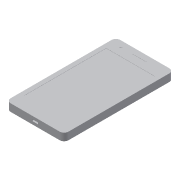
# Autodesk Inventor part: Galaxy S2
Saved by Autodesk Inventor 2013 (Build 170138000, 138)
## iProperties
Created: 2013-06-30
Part Number: Galaxy S2
Material: Allgemein
Document SubType Name: Modeling
Designer: Harald
Density: 1 g/cm^3
Author: Harald
Autodesk Inventor part; units mm, degrees
ref_plane "YZ Plane" through (0, 0, 0) normal (1, 0, 0) x (0, 1, 0)
ref_plane "XZ Plane" through (0, 0, 0) normal (0, 1, 0) x (-1, 0, 0)
ref_plane "XY Plane" through (0, 0, 0) normal (0, 0, 1) x (1, 0, 0)
sketch "Skizze1" plane through (0, 0, 0) normal (0, 0, 1) x (1, 0, 0)
  line L0 (0, 0) -> (66.1, 0)
  line L1 (66.1, 0) -> (66.1, 125.3)
  line L2 (66.1, 125.3) -> (0, 125.3)
  line L3 (0, 125.3) -> (0, 0)
  dimension "d0" = 66.1
  dimension "d1" = 125.3
  constraints: 8 end point, 2 parallel, 1 horizontal, 1 perpendicular
  measures "d0" distance of L2.end L1.end
  measures "d1" distance of L0.end L1.end
extrude "Extrusion1" add sketch "Skizze1" along normal blind 8.5
fillet "Rundung1" radius 5 1 edges at (66.1, 125.3, 4.25)
fillet "Rundung2" radius 5 1 edges at (0, 125.3, 4.25)
fillet "Rundung3" radius 5 1 edges at (0, 0, 4.25)
fillet "Rundung4" radius 5 1 edges at (66.1, 0, 4.25)
sketch "Skizze2" plane through (0, 0, 8.5) normal (0, 0, 1) x (1, 0, 0)
  line L0 (66.1, 5) -> (66.1, 120.3) projected
  line L1 (61.1, 125.3) -> (5, 125.3) projected
  line L2 (0, 120.3) -> (0, 5) projected
  line L3 (5.05, 109.15) -> (61.05, 109.15)
  line L4 (61.05, 109.15) -> (61.05, 16.15)
  line L5 (61.05, 16.15) -> (5.05, 16.15)
  line L6 (5.05, 16.15) -> (5.05, 109.15)
  point P0 (0, 0)
  dimension "d8" = 56
  dimension "d9" = 93
  dimension "d10" = 5.05
  dimension "d11" = 16.15
  constraints: 8 end point, 2 parallel, 1 horizontal, 1 perpendicular
  measures "d8" distance of L4.end L5.end
  measures "d9" distance of L3.end L4.end
  measures "d10" distance between parallel lines of L6 L2
  measures "d11" distance between parallel lines of L3 L1
sketch "Skizze3" plane through (0, 0, 8.5) normal (0, 0, 1) x (1, 0, 0)
  line L0 (66.1, 5) -> (66.1, 120.3) projected
  line L1 (61.1, 125.3) -> (5, 125.3) projected
  line L2 (0, 120.3) -> (0, 5) projected
  line L3 (5, 0) -> (61.1, 0) projected
  circle A0 centre (12, 118.6) radius 1.5
  line L4 (25.9, 119.7) -> (40.2, 119.7)
  arc A1 (40.2, 118.3) -> (40.2, 119.7) centre (40.2, 119) ccw
  line L5 (40.2, 118.3) -> (25.9, 118.3)
  arc A2 (25.9, 119.7) -> (25.9, 118.3) centre (25.9, 119) ccw
  point P0 (0, 0)
  dimension "d0" = 66.1
  dimension "d12" = 6.7
  dimension "d13" = 12
  dimension "d14" = 3
  dimension "d19" = 1.4
  dimension "d22" = 5.6
  dimension "d23" = 15.7
  dimension "d27" = 14.3
  dimension "d28" = 25.9
  constraints: 4 end point, 4 point on circle, 3 centre point, 2 parallel, 1 equal radius, 1 tangent, 1 vertical alignment
  measures "d12" distance from line of A0.centre L1
  measures "d13" distance from line of L2 A0.centre
  measures "d14" diameter of A0
  measures "d19" distance between parallel lines of L5 L4
  measures "d22" distance between parallel lines of L4 L1
  measures "d27" distance of A2.centre A1.centre
  measures "d28" distance from line of L0 A1.centre
extrude "Extrusion2" add sketch "Skizze3" along normal blind 0.2
extrude "Extrusion3" cut sketch "Skizze2" against normal blind 0.2
sketch "Skizze5" plane through (5, 0, 0) normal (0, -1, 0) x (1, 0, 0)
  line L0 (0, 8.5) -> (56.1, 8.5) projected
  line L1 (0, 0) -> (0, 8.5) projected
  line L2 (0, 0) -> (56.1, 0) projected
  line L3 (24.575, 5.15) -> (31.425, 5.15)
  line L4 (31.425, 5.15) -> (31.425, 3.35)
  line L5 (31.425, 3.35) -> (24.575, 3.35)
  line L6 (24.575, 3.35) -> (24.575, 5.15)
  line L7 (56.1, 8.5) -> (56.1, 0) projected
  line L8 (0, 8.5) -> (56.1, 8.5) projected
  line L9 (0, 0) -> (0, 8.5) projected
  line L10 (0, 0) -> (56.1, 0) projected
  point P0 (-5, 0)
  dimension "d33" = 6.85
  dimension "d34" = 1.8
  dimension "d35" = 24.575
  dimension "d36" = 3.35
  constraints: 8 end point, 2 parallel, 1 horizontal, 1 perpendicular
  measures "d33" distance of L4.end L5.end
  measures "d34" distance of L3.end L4.end
  measures "d35" distance between parallel lines of L6 L1
  measures "d36" distance between parallel lines of L2 L5
extrude "Extrusion4" cut sketch "Skizze5" against normal blind 2 contours L3 L4 L5 L6
equation "\"d10\" = -0.5 * d8 + 0.5 * d0"
equation "\"d11\" = -0.5 * d9 + 0.5 * d1"
equation "\"d28\" = 0.5 * d0 - 0.5 * d27"
equation "\"d35\" = -0.5 * d33 + 0.5 * d8"
